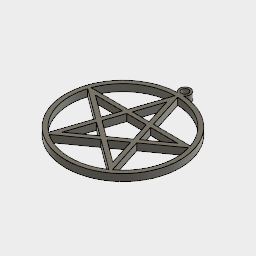
TEST9 (Autodesk Fusion 360 design; units mm, degrees)
Autodesk Fusion 360 part; units mm, degrees
sketch "草图1" plane through (0, 0, 0) normal (0, 1, 0) x (1, 0, 0)
  circle A0 centre (0, 0) radius 40.6099
  arc A1 (22.6638, -30.0143) -> (36.1396, 10.4131) centre (0, 0) ccw
  arc A2 (35.5488, 12.2796) -> (1.2643, 37.5886) centre (0, 0) ccw
  arc A3 (-21.5418, -30.8295) -> (21.0712, -31.153) centre (0, 0) ccw
  arc A4 (-0.6935, 37.6035) -> (-35.3582, 12.8179) centre (0, 0) ccw
  arc A5 (-35.9774, 10.9606) -> (-23.1169, -29.6667) centre (0, 0) ccw
  line L0 (-9.022, 12.618) -> (-35.3582, 12.8179)
  line L1 (-10.0195, 9.6255) -> (-29.3159, 9.772)
  line L2 (0.2346, 30.9008) -> (-5.8677, 12.5941)
  line L3 (-0.6935, 37.6035) -> (-9.022, 12.618)
  line L4 (0.2346, 30.9008) -> (6.0582, 12.5035)
  line L5 (35.5488, 12.2796) -> (9.2125, 12.4796)
  line L6 (6.0582, 12.5035) -> (-5.8677, 12.5941)
  line L7 (1.2643, 37.5886) -> (9.2125, 12.4796)
  line L8 (29.4609, 9.3258) -> (10.1644, 9.4723)
  line L9 (7.0102, 9.4962) -> (-6.8652, 9.6015)
  line L10 (13.7636, -1.8979) -> (29.4609, 9.3258)
  line L11 (14.7156, -4.9052) -> (36.1396, 10.4131)
  line L12 (7.0102, 9.4962) -> (11.1977, -3.7326)
  line L13 (12.1496, -6.7399) -> (17.9733, -25.1372)
  line L14 (10.1644, 9.4723) -> (13.7636, -1.8979)
  line L15 (14.7156, -4.9052) -> (22.6638, -30.0143)
  line L16 (17.9733, -25.1372) -> (2.4482, -13.6765)
  line L17 (21.0712, -31.153) -> (-0.1178, -15.5112)
  line L18 (-18.3528, -24.8614) -> (-2.6556, -13.6377)
  line L19 (-0.0896, -11.8031) -> (11.1977, -3.7326)
  line L20 (-21.5418, -30.8295) -> (-0.1178, -15.5112)
  line L21 (2.4482, -13.6765) -> (12.1496, -6.7399)
  line L22 (-6.8652, 9.6015) -> (-11.2531, -3.5621)
  line L23 (-12.2506, -6.5546) -> (-18.3528, -24.8614)
  line L24 (-2.6556, -13.6377) -> (-12.2506, -6.5546)
  line L25 (-14.7884, -4.6812) -> (-35.9774, 10.9606)
  line L26 (-0.0896, -11.8031) -> (-11.2531, -3.5621)
  line L27 (-13.7909, -1.6887) -> (-29.3159, 9.772)
  line L28 (-10.0195, 9.6255) -> (-13.7909, -1.6887)
  line L29 (-14.7884, -4.6812) -> (-23.1169, -29.6667)
extrude "拉伸1" add sketch "草图1" along normal blind 5 makes body 1
sketch "草图2" plane through (0, 0, 0) normal (0, 1, 0) x (1, 0, 0)
  circle A0 centre (58.5356, 21.3067) radius 4
  circle A1 centre (58.5356, 21.3067) radius 2.5
  dimension "d6" = 8
  dimension "d7" = 5
  measures "d6" diameter of A0
  measures "d7" diameter of A1
extrude "拉伸2" add sketch "草图2" along normal blind 5 separate body makes body 2
move_body "移动1" bodies 2 to x (1, 0, 0) y (0, 1, 0) z (0, 0, 1) at (-58.3, 0, -22.5)
combine "合并1" operation add target body 1 tool bodies 2
